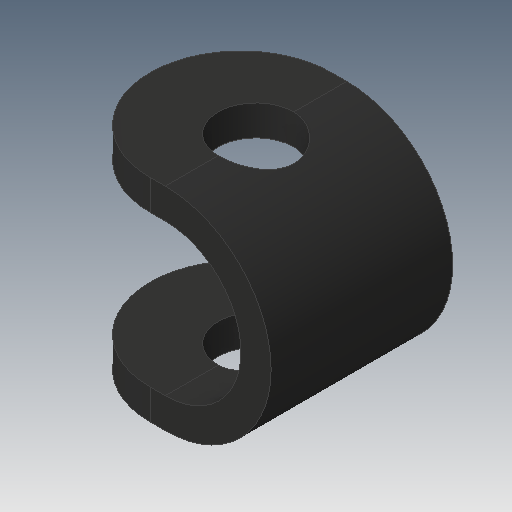
# Autodesk Inventor part: tip-protector
Saved by Autodesk Inventor 2017 (Build 210142000, 142)
## iProperties
Created: 2018-06-17
Part Number: tip-protector
Material: Rubber
Document SubType Name: Modeling
Designer: Luiz Gustavo
Density: 0.93 g/cm^3
Appearance: Rubber - Black
Mass: 0.601743 g
Surface Area: 8.70157 cm^2
Volume: 0.647036 cm^3
Author: Luiz Gustavo
Autodesk Inventor part; units mm, degrees
ref_plane "YZ Plane" through (0, 0, 0) normal (1, 0, 0) x (0, 1, 0)
ref_plane "XZ Plane" through (0, 0, 0) normal (0, 1, 0) x (-1, 0, 0)
ref_plane "XY Plane" through (0, 0, 0) normal (0, 0, 1) x (1, 0, 0)
sketch "Sketch4" plane through (0, 0, 0) normal (0, 0, 1) x (1, 0, 0)
  arc A0 (0, -5) -> (0, 5) centre (0, 0) ccw
  line L0 (0, -5) -> (-7, -5)
  line L1 (-5, -5) -> (-5, 5) construction
  line L2 (-7, 5) -> (0, 5)
  line L3 (0, 5) -> (0, -5) construction
  arc A1 (-5, 0) -> (0, -5) centre (0, 0) ccw construction
  arc A2 (0, 5) -> (-5, 0) centre (0, 0) ccw construction
  arc A3 (-5, -4.899) -> (-4.899, -5) centre (0, 0) ccw construction
  line L4 (0, -7) -> (-7, -7)
  line L5 (-7, -7) -> (-7, -5)
  line L6 (-7, 7) -> (0, 7)
  arc A4 (-7, 0) -> (-5, -4.899) centre (0, 0) ccw construction
  arc A5 (-5, 4.899) -> (-7, 0) centre (0, 0) ccw construction
  arc A6 (-4.899, 5) -> (-5, 4.899) centre (0, 0) ccw construction
  arc A7 (0, 7) -> (-4.899, 5) centre (0, 0) ccw construction
  arc A8 (-4.899, -5) -> (0, -7) centre (0, 0) ccw construction
  arc A9 (0, -7) -> (0, 7) centre (0, 0) ccw
  line L7 (-7, -5) -> (-7, 5) construction
  line L8 (-7, 5) -> (-7, 7)
  dimension "d14" = 10
  dimension "d15" = 2
  constraints: 26 point on circle, 20 tangent, 18 end point, 10 centre point, 8 point on line, 4 perpendicular, 3 coincident, 3 midpoint, 2 horizontal, 2 parallel
  measures "d14" diameter of A0
  measures "d15" radial gap between concentric circles of A3 A0
extrude "Extrusion4" add sketch "Sketch4" along normal mid plane 12
sketch "Sketch5" plane through (0, 0, 0) normal (0, 1, 0) x (-1, 0, 0)
  circle A0 centre (0, 0) radius 2.5
  dimension "d18" = 5
  constraints: 1 centre point, 1 coincident
  measures "d18" diameter of A0
extrude "Extrusion5" cut sketch "Sketch5" along normal through all both and the other way through all
fillet "Fillet1" radius 6 4 edges at (-7, 6, 6) (-7, 6, -6) (-7, -6, -6) (-7, -6, 6)
body "Solid3"
